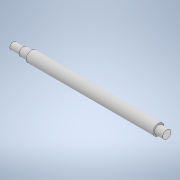
# Autodesk Inventor part: Eixo
Saved by Autodesk Inventor 2020.2 (Build 242310000, 310)
## iProperties
Created: 2020-11-25
Part Number: Eixo
Material: Genérico
Document SubType Name: Modeling
Designer: Ryanm
Density: 1 g/cm^3
Appearance: Padrão
Author: Ryanm
Autodesk Inventor part; units mm, degrees
ref_plane "YZ Plane" through (0, 0, 0) normal (1, 0, 0) x (0, 1, 0)
ref_plane "XZ Plane" through (0, 0, 0) normal (0, 1, 0) x (-1, 0, 0)
ref_plane "XY Plane" through (0, 0, 0) normal (0, 0, 1) x (1, 0, 0)
sketch "Esboço1" plane through (0, 0, 0) normal (0, 0, 1) x (1, 0, 0)
  line L0 (0, 0) -> (-6, 0)
  line L1 (-6, 0) -> (-6, 2)
  line L2 (-6, 2) -> (0, 2)
  line L3 (0, 2) -> (0, 0)
  line L4 (0, 0) -> (5, 0)
  line L5 (5, 0) -> (5, 2.5)
  line L6 (5, 2.5) -> (0, 2.5)
  line L7 (0, 2.5) -> (0, 0)
  line L8 (5, 0) -> (6, 0)
  line L9 (6, 0) -> (6, 3.25)
  line L10 (6, 3.25) -> (5, 3.25)
  line L11 (5, 3.25) -> (5, 0)
  line L12 (6, 0) -> (81, 0)
  line L13 (81, 0) -> (81, 3.25)
  line L14 (81, 3.25) -> (6, 3.25)
  line L15 (6, 3.25) -> (6, 0)
  line L16 (81, 0) -> (86, 0)
  line L17 (86, 0) -> (86, 2.5)
  line L18 (86, 2.5) -> (81, 2.5)
  line L19 (81, 2.5) -> (81, 0)
  dimension "d0" = 6
  dimension "d1" = 2
  dimension "d2" = 5
  dimension "d3" = 2.5
  dimension "d4" = 1
  dimension "d5" = 3.25
  dimension "d6" = 3.25
  dimension "d7" = 75
  dimension "d8" = 5
  dimension "d9" = 2.5
  constraints: 40 end point, 10 parallel, 5 horizontal, 5 perpendicular
  measures "d0" distance of L1.end L2.end
  measures "d1" distance of L0.end L1.end
  measures "d2" distance of L6.end L5.end
  measures "d3" distance of L5.end L4.end
  measures "d4" distance of L10.end L9.end
  measures "d5" distance of L9.end L8.end
  measures "d6" distance of L13.end L12.end
  measures "d7" distance of L13.end L14.end
  measures "d8" distance of L18.end L17.end
  measures "d9" distance of L17.end L16.end
revolve "Revolução1" add sketch "Esboço1" angle 360 about axis through (6, 0, 0) along (1, 0, 0)
